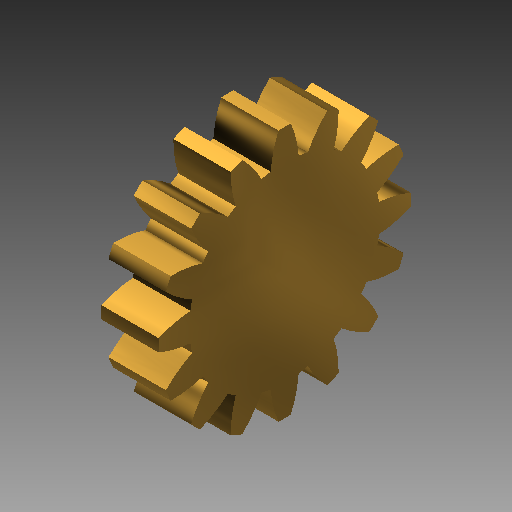
# Autodesk Inventor part: Shaft
Saved by Autodesk Inventor 2019 (Build 230136000, 136)
## iProperties
Created: 2017-05-31
Part Number: Shaft
Material: Brass, Soft Yellow
Document SubType Name: Modeling
Designer: Autodesk Inc.
Density: 8.47 g/cm^3
Appearance: Brass - Satin
CustomPartVersion: 1
Company: Autodesk Inc.
Author: Inventor
Autodesk Inventor part; units mm, degrees
ref_plane "Start Plane" through (0, 0, 0) normal (1, 0, 0) x (0, 1, 0)
ref_plane "XZ Plane" through (0, 0, 0) normal (0, 1, 0) x (-1, 0, 0)
ref_plane "XY Plane" through (0, 0, 0) normal (0, 0, 1) x (1, 0, 0)
sketch "Main Sketch" plane through (0, 0, 0) normal (0, 0, 1) x (1, 0, 0)
  line L0 (0, 0) -> (2.15, 0)
  line L1 (0, 0) -> (0, 4.916)
  line L2 (2.15, 4.916) -> (2.15, 0)
  line L3 (0, 4.916) -> (2.15, 4.916)
  dimension "d3" = 9.832
  constraints: 8 end point, 2 horizontal, 2 vertical
  measures "d3" diameter of L3 L0
revolve "Revolution1" add sketch "Main Sketch" angle 360 about axis through (0, 0, 0) along (1, 0, 0)
spur gear teeth "Spur Gear1" teeth 16 pitch diameter 8.4667 tip diameter 9.4551 root diameter 7.1437 face width 2.15 trims to tip circle yes start plane through (0, 0, 0) normal (-1, 0, 0) x (0, -1, 0)
body "Solid1"
